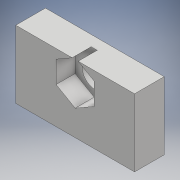
# Autodesk Inventor part: nutholder
Saved by Autodesk Inventor 2017 (Build 210142000, 142)
## iProperties
Created: 2017-12-20
Part Number: nutholder
Material: Generic
Document SubType Name: Modeling
Designer: will
Density: 1 g/cm^3
Appearance: Default
Author: will
Autodesk Inventor part; units mm, degrees
ref_plane "YZ Plane" through (0, 0, 0) normal (1, 0, 0) x (0, 1, 0)
ref_plane "XZ Plane" through (0, 0, 0) normal (0, 1, 0) x (-1, 0, 0)
ref_plane "XY Plane" through (0, 0, 0) normal (0, 0, 1) x (1, 0, 0)
sketch "Sketch1" plane through (0, 0, 0) normal (0, 1, 0) x (-1, 0, 0)
  line L0 (75.4269, 64.9582) -> (50.4269, 64.9582)
  line L1 (50.4269, 64.9582) -> (50.4269, 44.9582)
  line L2 (50.4269, 44.9582) -> (75.4269, 44.9582)
  line L3 (75.4269, 44.9582) -> (75.4269, 64.9582)
  line L4 (62.9269, 50.3394) -> (58.9269, 52.6488)
  line L5 (58.9269, 52.6488) -> (58.9269, 57.2676)
  line L6 (58.9269, 57.2676) -> (62.9269, 59.577)
  line L7 (62.9269, 59.577) -> (66.9269, 57.2676)
  line L8 (66.9269, 57.2676) -> (66.9269, 52.6488)
  line L9 (66.9269, 52.6488) -> (62.9269, 50.3394)
  line L10 (50.4269, 54.9582) -> (62.9269, 54.9582) construction
  line L11 (62.9269, 54.9582) -> (75.4269, 54.9582) construction
  point P0 (0, 0)
  dimension "d0" = 25
  dimension "d1" = 20
  dimension "d2" = 8
  constraints: 24 end point, 2 horizontal, 2 midpoint, 2 parallel, 1 collinear, 1 perpendicular, 1 vertical, 13 other
  measures "d0" distance of L2.end L1.end
  measures "d1" distance of L1.end L0.end
  measures "d2" distance between parallel lines of L6 L9
extrude "Extrusion1" add sketch "Sketch1" along normal blind 6.25
sketch "Sketch2" plane through (0, 6.25, 0) normal (0, 1, 0) x (1, 0, 0)
  line L0 (-62.9269, -59.577) -> (-66.9269, -57.2676) projected
  line L1 (-66.9269, -57.2676) -> (-66.9269, -52.6488) projected
  line L2 (-66.9269, -52.6488) -> (-62.9269, -50.3394) projected
  line L3 (-62.9269, -50.3394) -> (-58.9269, -52.6488) projected
  line L4 (-58.9269, -57.2676) -> (-62.9269, -59.577) projected
  line L5 (-58.9269, -52.6488) -> (-58.9269, -57.2676) projected
  circle A0 centre (-62.6988, -54.542) radius 2.75
  point P0 (0, 0)
  dimension "d5" = 5.5
  constraints: 1 centre point
  measures "d5" diameter of A0
extrude "Extrusion2" add sketch "Sketch2" against normal blind 2.25
sketch "Sketch3" plane through (-75.4269, 0, 64.9582) normal (0, 0, 1) x (1, 0, 0)
  line L0 (0, 0) -> (25, 0) projected
  line L1 (25, 0) -> (25, 6.25) projected
  line L2 (0, 6.25) -> (25, 6.25) projected
  line L3 (0, 0) -> (0, 6.25) projected
  point P0 (75.4269, 0)
extrude "Extrusion3" cut sketch "Sketch3" against normal blind 5.75
body "Solid1"
